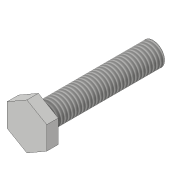
# Autodesk Inventor part: Counterweight Bolt
Saved by Autodesk Inventor 2018.3 (Build 223284000, 284)
## iProperties
Created: 2019-01-07
Part Number: Counterweight Bolt
Material: Generic
Document SubType Name: Modeling
Designer: aye06091
Mass: 10.7049 g
Surface Area: 38.5549 cm^2
Volume: 10.7049 cm^3
Density: 1 g/cm^3
Appearance: Default
Author: aye06091
Autodesk Inventor part; units mm, degrees
ref_plane "YZ Plane" through (0, 0, 0) normal (1, 0, 0) x (0, 1, 0)
ref_plane "XZ Plane" through (0, 0, 0) normal (0, 1, 0) x (-1, 0, 0)
ref_plane "XY Plane" through (0, 0, 0) normal (0, 0, 1) x (1, 0, 0)
sketch "Sketch1" plane through (0, 0, 0) normal (0, 0, 1) x (1, 0, 0)
  line L0 (0, 12.7) -> (10.9985, 6.35)
  line L1 (10.9985, 6.35) -> (10.9985, -6.35)
  line L2 (10.9985, -6.35) -> (0, -12.7)
  line L3 (0, -12.7) -> (-10.9985, -6.35)
  line L4 (-10.9985, -6.35) -> (-10.9985, 6.35)
  line L5 (-10.9985, 6.35) -> (0, 12.7)
  point P0 (0, 0)
  point P1 (0, 0)
  dimension "d3" = 25.4
  constraints: 12 end point, 1 coincident, 13 other
  measures "d3" distance of L2.end L0.start
extrude "Extrusion1" add sketch "Sketch1" against normal blind 6.35
sketch "Sketch2" plane through (0, 0, -6.35) normal (0, 0, -1) x (-1, 0, 0)
  circle A0 centre (0, 0) radius 6.35
  dimension "d2" = 12.7
  constraints: 1 centre point, 1 coincident
  measures "d2" diameter of A0
extrude "Extrusion2" add sketch "Sketch2" along normal blind 63.5
thread "Thread1" size "1/2-13 UNC" class "2A" standard "ANSI Unified Screw Threads" full length
body "Solid1"
